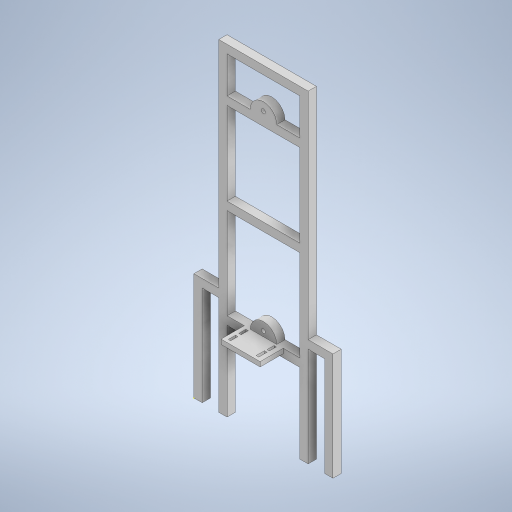
# Autodesk Inventor part: Frame_final
Saved by Autodesk Inventor 2023 (Build 270158000, 158)
## iProperties
Created: 2023-02-14
Part Number: Frame_final
Material: Generic
Document SubType Name: Modeling
Designer: 91882
Density: 1 g/cm^3
Appearance: Default
Author: 91882
Autodesk Inventor part; units mm, degrees
ref_plane "YZ Plane" through (0, 0, 0) normal (1, 0, 0) x (0, 1, 0)
ref_plane "XZ Plane" through (0, 0, 0) normal (0, 1, 0) x (-1, 0, 0)
ref_plane "XY Plane" through (0, 0, 0) normal (0, 0, 1) x (1, 0, 0)
sketch "Sketch1" plane through (0, 0, 0) normal (0, 0, 1) x (1, 0, 0)
  point P0 (0, 0)
sketch "Sketch2" plane through (0, 0, 0) normal (0, 0, 1) x (1, 0, 0)
  line L0 (0, 0) -> (25, 0)
  line L1 (25, 0) -> (25, 300)
  line L2 (25, 300) -> (75, 300)
  line L3 (75, 300) -> (75, 0)
  line L4 (75, 0) -> (100, 0)
  line L5 (100, 0) -> (100, 240)
  line L6 (100, 240) -> (320, 240)
  line L7 (320, 240) -> (320, 0)
  line L8 (320, 0) -> (345, 0)
  line L9 (345, 0) -> (345, 300)
  line L10 (345, 300) -> (395, 300)
  line L11 (395, 300) -> (395, 0)
  line L12 (395, 0) -> (420, 0)
  line L13 (420, 0) -> (420, 325)
  line L14 (420, 325) -> (345, 325)
  line L15 (345, 325) -> (345, 975)
  line L16 (345, 975) -> (75, 975)
  line L17 (75, 975) -> (75, 325)
  line L18 (75, 325) -> (0, 325)
  line L19 (0, 325) -> (0, 0)
  dimension "d0" = 25
  dimension "d1" = 300
  dimension "d2" = 50
  dimension "d3" = 300
  dimension "d4" = 25
  dimension "d5" = 240
  dimension "d6" = 220
  dimension "d7" = 240
  dimension "d8" = 25
  dimension "d9" = 300
  dimension "d10" = 50
  dimension "d11" = 300
  dimension "d12" = 25
  dimension "d13" = 325
  dimension "d14" = 75
  dimension "d15" = 650
  dimension "d16" = 270
  dimension "d17" = 650
  dimension "d18" = 75
  constraints: 40 end point, 13 point on line, 5 perpendicular, 1 horizontal, 1 parallel
  measures "d0" distance of L0.start L0.end
  measures "d1" distance of L0.end L1.end
  measures "d2" distance of L1.end L2.end
  measures "d3" distance of L2.end L3.end
  measures "d4" distance of L3.end L4.end
  measures "d5" distance of L4.end L5.end
  measures "d6" distance of L5.end L6.end
  measures "d7" distance of L6.end L7.end
  measures "d8" distance of L7.end L8.end
  measures "d9" distance of L8.end L9.end
  measures "d10" distance of L9.end L10.end
  measures "d11" distance of L10.end L11.end
  measures "d12" distance of L11.end L12.end
  measures "d13" distance of L12.end L13.end
  measures "d14" distance of L13.end L14.end
  measures "d15" distance of L14.end L15.end
  measures "d16" distance of L15.end L16.end
  measures "d17" distance of L16.end L17.end
  measures "d18" distance of L17.end L18.end
sketch "Sketch3" plane through (0, 0, 0) normal (0, 0, 1) x (1, 0, 0)
  line L0 (100, 950) -> (320, 950)
  line L1 (320, 950) -> (320, 840)
  line L2 (320, 840) -> (100, 840)
  line L3 (100, 840) -> (100, 950)
  line L4 (100, 815) -> (320, 815)
  line L5 (320, 815) -> (320, 565)
  line L6 (320, 565) -> (100, 565)
  line L7 (100, 565) -> (100, 815)
  line L8 (100, 540) -> (320, 540)
  line L9 (320, 540) -> (320, 265)
  line L10 (320, 265) -> (100, 265)
  line L11 (100, 265) -> (100, 540)
  point P0 (0, 0)
  dimension "d19" = 220
  dimension "d20" = 110
  dimension "d21" = 220
  dimension "d22" = 250
  dimension "d23" = 220
  dimension "d24" = 275
  constraints: 24 end point, 6 parallel, 3 horizontal, 3 perpendicular, 1 point on line
  measures "d19" distance of L1.end L2.end
  measures "d20" distance of L0.end L1.end
  measures "d21" distance of L5.end L6.end
  measures "d22" distance of L4.end L5.end
  measures "d23" distance of L9.end L10.end
  measures "d24" distance of L8.end L9.end
extrude "Extrusion1" add sketch "Sketch2" along normal blind 25
extrude "Extrusion2" cut sketch "Sketch3" along normal through all
sketch "Sketch4" plane through (0, 0, 25) normal (0, 0, 1) x (1, 0, 0)
  line L0 (100, 840) -> (320, 840) projected
  arc A0 (250, 840) -> (170, 840) centre (210, 840) ccw
  point P0 (0, 0)
  constraints: 2 point on circle, 1 centre point, 1 midpoint, 1 point on line
extrude "Extrusion3" add sketch "Sketch4" against normal blind 25
sketch "Sketch5" plane through (0, 0, 25) normal (0, 0, 1) x (1, 0, 0)
  point P0 (0, 0)
sketch "Sketch6" plane through (0, 0, 25) normal (0, 0, 1) x (1, 0, 0)
  line L0 (320, 265) -> (100, 265) projected
  arc A0 (250, 265) -> (170, 265) centre (210, 265) ccw
  point P0 (0, 0)
  dimension "d31" = 40
  constraints: 2 point on circle, 1 centre point, 1 midpoint, 1 point on line
  measures "d31" radius of A0
extrude "Extrusion4" add sketch "Sketch6" against normal blind 25
sketch "Sketch7" plane through (0, 0, 25) normal (0, 0, 1) x (1, 0, 0)
  line L0 (170, 265) -> (100, 265) projected
  line L1 (152, 265) -> (270, 265)
  line L2 (270, 265) -> (270, 251)
  line L3 (270, 251) -> (152, 251)
  line L4 (152, 251) -> (152, 265)
  point P0 (0, 0)
  constraints: 8 end point, 2 parallel, 1 horizontal, 1 perpendicular, 1 point on line
extrude "Extrusion5" add sketch "Sketch7" along normal blind 70
sketch "Sketch8" plane through (100, 265, 25) normal (0, 1, 0) x (1, 0, 0)
  point P0 (-100, 25)
sketch "Sketch9" plane through (100, 265, 25) normal (0, 1, 0) x (1, 0, 0)
  line L0 (64, -7) -> (71, -7)
  line L1 (71, -7) -> (71, -28)
  line L2 (71, -28) -> (64, -28)
  line L3 (64, -28) -> (64, -7)
  line L4 (64, -38) -> (71, -38)
  line L5 (71, -38) -> (71, -60)
  line L6 (71, -60) -> (64, -60)
  line L7 (64, -60) -> (64, -38)
  line L8 (149, -7) -> (156, -7)
  line L9 (156, -7) -> (156, -28)
  line L10 (156, -28) -> (149, -28)
  line L11 (149, -28) -> (149, -7)
  line L12 (148, -35) -> (156, -35)
  line L13 (156, -35) -> (156, -60)
  line L14 (156, -60) -> (148, -60)
  line L15 (148, -60) -> (148, -35)
  point P0 (-100, 25)
  constraints: 32 end point, 8 parallel, 6 point on line, 4 horizontal, 4 perpendicular
extrude "Extrusion6" cut sketch "Sketch9" against normal through all
sketch "Sketch10" plane through (0, 0, 25) normal (0, 0, 1) x (1, 0, 0)
  circle A0 centre (210, 280) radius 6
  point P0 (0, 0)
  dimension "d38" = 12
  constraints: 1 centre point
  measures "d38" diameter of A0
sketch "Sketch11" plane through (0, 0, 25) normal (0, 0, 1) x (1, 0, 0)
  circle A0 centre (210, 855) radius 6
  point P0 (0, 0)
  dimension "d39" = 12
  constraints: 1 centre point
  measures "d39" diameter of A0
extrude "Extrusion7" cut sketch "Sketch11" against normal through all
extrude "Extrusion8" cut sketch "Sketch10" against normal through all
body "Solid1"
